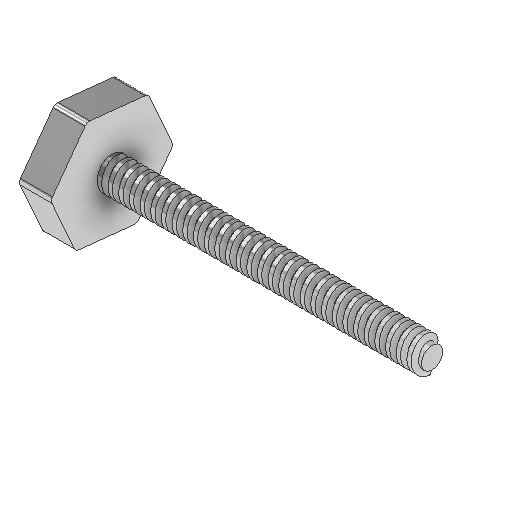
# Autodesk Inventor part: Screw
Saved by Autodesk Inventor 2026.2 (Build 302298000, 298)
## iProperties
Created: 2026-01-29
Part Number: Screw
Material: Generic
Document SubType Name: Modeling
Designer: andyeske
Density: 1 g/cm^3
Appearance: Default
Author: andyeske
Autodesk Inventor part; units mm, degrees
ref_plane "YZ Plane" through (0, 0, 0) normal (1, 0, 0) x (0, 1, 0)
ref_plane "XZ Plane" through (0, 0, 0) normal (0, 1, 0) x (-1, 0, 0)
ref_plane "XY Plane" through (0, 0, 0) normal (0, 0, 1) x (1, 0, 0)
sketch "Sketch1" plane through (0, 0, 0) normal (0, 0, 1) x (1, 0, 0)
  line L0 (0, 0) -> (-76.2, 0)
  line L1 (0, 0) -> (0, -2.54)
  line L2 (0, -2.54) -> (-76.2, -2.54)
  line L3 (-76.2, 0) -> (-76.2, -2.54)
  line L4 (-2.032, -2.54) -> (-1.524, -3.81)
  line L5 (-1.524, -3.81) -> (-0.508, -3.81)
  line L6 (-0.508, -3.81) -> (0, -2.54)
  dimension "d0" = 76.2
  dimension "d1" = 2.54
  dimension "d2" = 2.032
  dimension "d3" = 0.508
  dimension "d4" = 1.27
  constraints: 14 end point, 2 horizontal, 2 vertical, 1 equal length, 1 perpendicular, 1 point on line
  measures "d0" distance of L0.start L0.end
  measures "d1" distance of L0.end L2.end
  measures "d2" distance of L4.start L1.end
  measures "d3" horizontal distance of L4.end L4.start
  measures "d4" vertical distance of L1.end L5.end
revolve "Revolution1" add sketch "Sketch1" angle 360 about axis through (0, 0, 0) along (-1, 0, 0) contours L1 L2 L3 L0
sketch "Sketch2" plane through (0, 0, 0) normal (0, 0, 1) x (1, 0, 0)
  line L0 (-2.032, -2.54) -> (-1.524, -3.81) projected
  line L1 (-1.524, -3.81) -> (-0.508, -3.81) projected
  line L2 (-0.508, -3.81) -> (0, -2.54) projected
  line L3 (-2.032, -2.54) -> (0, -2.54)
  line L4 (0, -2.54) -> (-76.2, -2.54) projected
  point P0 (0, 0)
  constraints: 2 end point, 1 collinear
coil "Coil1" sketch "Sketch2" operation add axis through (-38.1, 0, 0) along (-1, 0, 0) pitch 2.54 turns 30 hand right
sketch "Sketch3" plane through (-76.2, 0, 0) normal (-1, 0, 0) x (0, -0.809, 0.5878)
  line L0 (7.3323, 12.7) -> (14.6647, 0)
  line L1 (14.6647, 0) -> (7.3323, -12.7)
  line L2 (7.3323, -12.7) -> (-7.3323, -12.7)
  line L3 (-7.3323, -12.7) -> (-14.6647, 0)
  line L4 (-14.6647, 0) -> (-7.3323, 12.7)
  line L5 (-7.3323, 12.7) -> (7.3323, 12.7)
  point P0 (0, 0)
  point P1 (0, 0)
  dimension "d18" = 25.4
  constraints: 12 end point, 1 coincident, 1 horizontal, 13 other
  measures "d18" distance between parallel lines of L5 L2
extrude "Extrusion1" add sketch "Sketch3" along normal blind 7.62
fillet "Fillet1" radius 1.27 6 edges at (-80.01, -1.5329, -14.5844) (-80.01, -13.3969, -5.9647) (-80.01, 11.864, -8.6197) (-80.01, 13.3969, 5.9647) (-80.01, 1.5329, 14.5844) (-80.01, -11.864, 8.6197)
equation "\"d0\" = Height"
equation "\"d1\" = 0.5 * Coil_Dia"
equation "\"d6\" = Pitch"
equation "\"d18\" = Head_Dia"
equation "\"d15\" = 0.1 * Height"
equation "\"Height\" = 76.2"
equation "\"Head_Dia\" = 25.4"
equation "\"Coil_Dia\" = 5.08"
equation "\"Pitch\" = 2.54"
body "Solid1"
